Autodesk Fusion 360 part; units mm, degrees
(part 2 of 2)
  spline S254 degree 3 poles (10.2703, -7.3178) (9.2938, -7.3178) (9.3929, -7.1693) (9.499, -8.45) knots 0 0 0 0 1 1 1 1
  spline S255 degree 3 poles (9.499, -8.45) (9.5698, -9.3133) (9.6476, -10.2261) (9.8245, -12.3065) knots 0 0 0 0 1 1 1 1
  spline S256 degree 3 poles (9.8245, -12.3065) (9.8811, -13.007) (9.959, -13.934) (9.9944, -14.3585) knots 0 0 0 0 1 1 1 1
  spline S257 degree 3 poles (9.9944, -14.3585) (10.1783, -16.6512) (10.2845, -17.9178) (10.3199, -18.1301) knots 0 0 0 0 1 1 1 1
  line L89 (10.3199, -18.1301) -> (10.3552, -18.3565)
  line L90 (10.3552, -18.3565) -> (11.36, -18.3565)
  line L91 (11.36, -18.3565) -> (12.3648, -18.3565)
  line L92 (12.3648, -18.3565) -> (12.7045, -17.6843)
  spline S258 degree 3 poles (11.4945, -13.7783) (11.445, -12.7735) (11.4096, -11.8182) (11.4096, -11.6555) knots 0 0 0 0 1 1 1 1
  line L93 (11.4096, -11.6555) -> (11.4096, -11.3512)
  line L94 (11.4096, -11.3512) -> (12.3012, -11.3512)
  spline S259 degree 3 poles (12.3012, -11.3512) (13.1149, -11.3512) (13.1857, -11.3583) (13.1644, -11.4786) knots 0 0 0 0 1 1 1 1
  spline S260 degree 3 poles (13.1644, -11.4786) (13.1291, -11.6979) (11.6572, -15.5968) (11.6148, -15.5968) knots 0 0 0 0 1 1 1 1
  spline S261 degree 3 poles (11.6148, -15.5968) (11.5936, -15.5968) (11.5369, -14.776) (11.4945, -13.7783) knots 0 0 0 0 1 1 1 1
extrude "Extrude7" cut sketch "Sketch9" against normal blind 2 contours S0 S1 S2 S3 S4 S5 S6 S7 S8 S9 S10 S11 S12 S13 S14 S15 S16 S17 S18 S19 S20 S21 S22 S23 S24 S25 S26 S27 S28 L5 L6 S29 | S174 L29 L30 S175 L31 L32 L33 L34 S176 S177 | L35 L36 L37 L38 S178 L39 L40 S179 S180 S181 S182 | L41 L42 S183 S184 S185 L43 L44 S186 S187 S188 S189 S190 L45 L46 L47 L48 S191 S192 L49 L50 L51 L52 S193 S194 S195 S196 L53 L54 S197 S198 S199 S200 S201 L55 L56 | S223 S224 L73 L74 S225 S226 S227 S228 S229 L75 L76 L77 L78 S230 S231 S232 S233 S234 S235 S236 L79 L80 | S245 S246 S247 S248 S249 S250 S251 S252 L83 L84 L85 L86 S253 L87 L88 S254 S255 S256 S257 L89 L90 L91 L92
sketch "Sketch10" plane through (0, 0, 4.5) normal (0, 0, 1) x (-1, 0, 0)
  arc A0 (0, -1.5) -> (-1.5, 0) centre (-1.5, -1.5) ccw
  line L0 (-1.5, 0) -> (-56.5, 0)
  arc A1 (-56.5, 0) -> (-72, -15.5) centre (-56.5, -15.5) ccw
  line L1 (-72, -15.5) -> (-72, -32)
  line L2 (-72, -32) -> (-72, -33)
  arc A2 (-72, -33) -> (-57, -48) centre (-57, -33) ccw
  line L3 (-57, -48) -> (-56, -48)
  line L4 (-56, -48) -> (-16, -48)
  line L5 (-16, -48) -> (-15, -48)
  arc A3 (-15, -48) -> (0, -33) centre (-15, -33) ccw
  line L6 (0, -33) -> (0, -32)
  line L7 (0, -32) -> (0, -1.5)
  arc A4 (-41.5, -45) -> (-29, -32.5) centre (-41.5, -32.5) ccw
  line L8 (-41.5, -45) -> (-56.5, -45)
  arc A5 (-69, -32.5) -> (-56.5, -45) centre (-56.5, -32.5) ccw
  line L9 (-69, -32.5) -> (-69, -15.5)
  arc A6 (-56.5, -3) -> (-69, -15.5) centre (-56.5, -15.5) ccw
  line L10 (-56.5, -3) -> (-41.5, -3)
  arc A7 (-29, -15.5) -> (-41.5, -3) centre (-41.5, -15.5) ccw
  line L11 (-29, -15.5) -> (-29, -32.5)
  line L12 (-4, -4) -> (-24, -4) construction
  line L13 (-24, -4) -> (-24, -14) construction
  line L14 (-24, -14) -> (-4, -14) construction
  line L15 (-4, -14) -> (-4, -4) construction
  dimension "d100" = 7
  dimension "d101" = 4
  dimension "d102" = 4
  dimension "d103" = 20
  dimension "d104" = 10
  text T0 "Inky" font "Arial" height 7 align centre top in box 20 x 10 at (-4, -4) x (-1, 0) y (0, -1) spacing 1
  constraint horizontal L12
  measures "d101" distance of L0 L12
  measures "d102" distance of L7 L15
  measures "d103" distance of L13 L15
  measures "d104" distance of L12 L14
extrude "Extrude8" cut sketch "Sketch10" against normal blind 0.5 text T0
equation "d71 = 8.3 mm + 1.7 mm"
equation "d82 = 12.5 mm + 3 mm"
